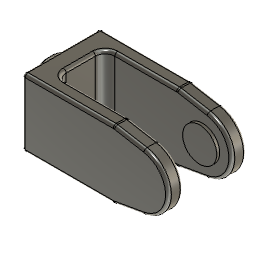
link4 (Autodesk Fusion 360 design; units mm, degrees)
part number: 2025-12-13-23-07-16-757
Autodesk Fusion 360 part; units mm, degrees
sketch "Sketch1" plane through (0, 0, 0) normal (0, 1, 0) x (1, 0, 0)
  line L0 (0, 0) -> (0, -70)
  line L1 (0, -70) -> (94.2683, -70)
  line L2 (94.2683, -70) -> (125.2094, -64.5442)
  arc A0 (125.2094, -64.5442) -> (125.2094, -5.4558) centre (120, -35) ccw
  line L3 (125.2094, -5.4558) -> (94.2683, 0)
  line L4 (94.2683, 0) -> (0, 0)
  dimension "d1" = 70
  dimension "d2" = 30
  dimension "d3" = 170
  dimension "d4" = 120
  constraint coincident L0.start L4.end
  constraint vertical L0
  constraint perpendicular L0 L1
  constraint equal L2 L3
  constraint equal L1 L4
  constraint horizontal L4
  constraint tangent L2 A0
  constraint tangent A0 L3
  measures "d1" distance of L0.start L0.end
  measures "d2" radius of A0
  measures "d3" angle of L3 L4
  measures "d4" horizontal distance of L0.start A0.centre
extrude "Extrude1" add sketch "Sketch1" along normal mid plane 80
sketch "Sketch2" plane through (0, 0, 70) normal (0, 0, 1) x (-1, 0, 0)
  line L0 (-94.2683, 40) -> (-94.2683, -40)
  line L1 (-94.2683, -40) -> (0, -40)
  line L2 (0, -40) -> (0, 40)
  line L3 (0, 40) -> (-94.2683, 40)
  line L4 (-20, -25) -> (-190, -25)
  line L5 (-190, -25) -> (-190, 25)
  line L6 (-190, 25) -> (-20, 25)
  line L7 (-20, 25) -> (-20, -25)
  dimension "d7" = 15
  dimension "d8" = 15
  dimension "d9" = 170
  dimension "d10" = 20
  constraint horizontal L4
  constraint vertical L5
  constraint horizontal L6
  constraint vertical L7
  measures "d7" distance of L1 L4.start
  measures "d8" distance of L3 L6
  measures "d9" distance of L5.end L6.end
  measures "d10" distance of L2 L4.start
extrude "Extrude2" cut sketch "Sketch2" against normal through all contours L0 L4 L6 L7 | L0 L4 L5 L6
sketch "Sketch3" plane through (0, 25, 0) normal (0, -1, 0) x (1, 0, 0)
  line L0 (125.2094, 64.5442) -> (94.2683, 70)
  line L1 (94.2683, 70) -> (20, 70)
  line L2 (20, 70) -> (20, 0)
  line L3 (20, 0) -> (94.2683, 0)
  line L4 (94.2683, 0) -> (125.2094, 5.4558)
  arc A0 (125.2094, 5.4558) -> (125.2094, 64.5442) centre (120, 35) ccw
  circle A1 centre (120, 35) radius 17.5
  dimension "d12" = 35
  constraint concentric A0 A1
  measures "d12" diameter of A1
extrude "Extrude3" add sketch "Sketch3" along normal blind 3 contours A1
mirror "Mirror1" about plane through (0, 0, 0) normal (0, 1, 0) of "Extrude3"
sketch "Sketch4" plane through (0, 0, 0) normal (-1, 0, 0) x (0, -1, 0)
  line L0 (40, 70) -> (-40, 70)
  line L1 (-40, 70) -> (-40, 0)
  line L2 (-40, 0) -> (40, 0)
  line L3 (40, 0) -> (40, 70)
  circle A0 centre (0, 35) radius 25
  line L4 (0, 35) -> (-40, 35) construction
  line L5 (0, 35) -> (0, 0) construction
  dimension "d17" = 50
  constraint coincident A0.centre L4.start
  constraint midpoint L1 L4.end
  constraint coincident L5.end origin
  constraint perpendicular L2 L5
  constraint horizontal L4
  measures "d17" diameter of A0
extrude "Extrude4" add sketch "Sketch4" along normal blind 10 contours A0
sketch "Sketch5" plane through (-10, 0, 0) normal (-1, 0, 0) x (0, -1, 0)
  circle A0 centre (0, 35) radius 25
  circle A1 centre (0, 35) radius 22
  dimension "d20" = -3
extrude "Extrude5" add sketch "Sketch5" along normal blind 3 contours A1
fillet "Fillet1" radius 10 6 edges at (20, 25, 35) (20, -25, 35) (94.2683, 32.5, 70) (94.2683, -32.5, 70) (94.2683, -32.5, 0) (94.2683, 32.5, 0)
fillet "Fillet2" radius 3 39 edges at (0, 0, 70) (46.6967, 40, 70) (94.2649, 40, 69.9619) (110.1696, 40, 67.1962) (150, 40, 35) (110.1696, 40, 2.8038) (94.2649, 40, 0.0381) (46.6967, 40, 0) (46.6967, -40, 0) (94.2649, -40, 0.0381) (110.1696, -40, 2.8038) (150, -40, 35) (110.1696, -40, 67.1962) (94.2649, -40, 69.9619) (46.6967, -40, 70) (22.9289, -22.0711, 70) (20, 0, 70) (22.9289, 22.0711, 70) (61.6967, 25, 70) (94.2649, 25, 69.9619) (110.1696, 25, 67.1962) (150, 25, 35) (110.1696, 25, 2.8038) (94.2649, 25, 0.0381) (61.6967, 25, 0) (22.9289, 22.0711, 0) (20, 0, 0) (22.9289, -22.0711, 0) (61.6967, -25, 0) (94.2649, -25, 0.0381) (110.1696, -25, 2.8038) (150, -25, 35) (110.1696, -25, 67.1962) (94.2649, -25, 69.9619) (61.6967, -25, 70) (0, 23.3082, 44.0404) (0, 40, 35) (0, -40, 35) (0, 0, 0)
